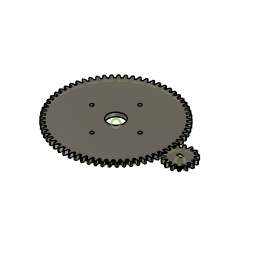
Gears v6 (Autodesk Fusion 360 design; units mm, degrees)
description: Spur Gear; Module: 2.0; Num Teeth: 15; Pressure Angle: 20.0; Backlash: 0.15 mm
description: Spur Gear; Module: 2.0; Num Teeth: 65; Pressure Angle: 20.0; Backlash: 0.15 mm
Autodesk Fusion 360 part; units mm, degrees
(part 1 of 8)
sketch "Sketch1" plane through (0, 0, 0) normal (0, 0, 1) x (1, 0, 0) in component "Spur Gear (15 teeth)"
  circle A0 centre (0, 0) radius 12.5492
extrude "Extrude1" add sketch "Sketch1" along normal blind 5 makes body 1 in component "Spur Gear (15 teeth)"
sketch "Sketch2" plane through (0, 0, 0) normal (0, 0, 1) x (1, 0, 0) in component "Spur Gear (15 teeth)"
  spline S0 degree 5 poles (13.9988, -1.6471) (14.0073, -1.6481) (14.0244, -1.6499) (14.05, -1.6517) (14.0843, -1.6528) (14.1272, -1.6522) (14.1702, -1.6502) (14.2133, -1.6473) (14.2564, -1.644) (14.2995, -1.6403) (14.3427, -1.6363) (14.3859, -1.6318) (14.4291, -1.6268) (14.4723, -1.621) (14.5156, -1.6146) (14.5589, -1.6075) (14.6022, -1.5999) (14.6454, -1.5918) (14.6887, -1.5833) (14.732, -1.5744) (14.7753, -1.5652) (14.8186, -1.5555) (14.8619, -1.5454) (14.9052, -1.5349) (14.9484, -1.524) (14.9917, -1.5126) (15.0349, -1.5009) (15.0782, -1.4887) (15.1214, -1.4762) (15.1646, -1.4634) (15.2077, -1.4502) (15.2509, -1.4366) (15.294, -1.4227) (15.3372, -1.4084) (15.3803, -1.3938) (15.4233, -1.3789) (15.4664, -1.3636) (15.5094, -1.348) (15.5524, -1.332) (15.5953, -1.3157) (15.6383, -1.2991) (15.6811, -1.2822) (15.724, -1.265) (15.7668, -1.2475) (15.8096, -1.2296) (15.8524, -1.2115) (15.8951, -1.193) (15.9378, -1.1743) (15.9804, -1.1552) (16.023, -1.1359) (16.0655, -1.1162) (16.108, -1.0963) (16.1505, -1.0761) (16.1929, -1.0556) (16.2353, -1.0348) (16.2776, -1.0137) (16.3199, -0.9924) (16.3621, -0.9707) (16.4043, -0.9488) (16.4464, -0.9266) (16.4885, -0.9042) (16.5305, -0.8814) (16.5725, -0.8584) (16.6144, -0.8351) (16.6562, -0.8116) (16.698, -0.7878) (16.7398, -0.7637) (16.7814, -0.7394) (16.8231, -0.7148) (16.8646, -0.6899) (16.9061, -0.6648) (16.9393, -0.6445) (16.9641, -0.6292) (16.9806, -0.6189) (16.9889, -0.6138) knots 0 0 0 0 0 0 0.01428571 0.02857143 0.04285714 0.05714286 0.07142857 0.08571429 0.1 0.11428571 0.12857143 0.14285714 0.15714286 0.17142857 0.18571429 0.2 0.21428571 0.22857143 0.24285714 0.25714286 0.27142857 0.28571429 0.3 0.31428571 0.32857143 0.34285714 0.35714286 0.37142857 0.38571429 0.4 0.41428571 0.42857143 0.44285714 0.45714286 0.47142857 0.48571429 0.5 0.51428571 0.52857143 0.54285714 0.55714286 0.57142857 0.58571429 0.6 0.61428571 0.62857143 0.64285714 0.65714286 0.67142857 0.68571429 0.7 0.71428571 0.72857143 0.74285714 0.75714286 0.77142857 0.78571429 0.8 0.81428571 0.82857143 0.84285714 0.85714286 0.87142857 0.88571429 0.9 0.91428571 0.92857143 0.94285714 0.95714286 0.97142857 0.98571429 1 1 1 1 1 1
  spline S1 degree 5 poles (13.9988, 1.6471) (14.0073, 1.6481) (14.0244, 1.6499) (14.05, 1.6517) (14.0843, 1.6528) (14.1272, 1.6522) (14.1702, 1.6502) (14.2133, 1.6473) (14.2564, 1.644) (14.2995, 1.6403) (14.3427, 1.6363) (14.3859, 1.6318) (14.4291, 1.6268) (14.4723, 1.621) (14.5156, 1.6146) (14.5589, 1.6075) (14.6022, 1.5999) (14.6454, 1.5918) (14.6887, 1.5833) (14.732, 1.5744) (14.7753, 1.5652) (14.8186, 1.5555) (14.8619, 1.5454) (14.9052, 1.5349) (14.9484, 1.524) (14.9917, 1.5126) (15.0349, 1.5009) (15.0782, 1.4887) (15.1214, 1.4762) (15.1646, 1.4634) (15.2077, 1.4502) (15.2509, 1.4366) (15.294, 1.4227) (15.3372, 1.4084) (15.3803, 1.3938) (15.4233, 1.3789) (15.4664, 1.3636) (15.5094, 1.348) (15.5524, 1.332) (15.5953, 1.3157) (15.6383, 1.2991) (15.6811, 1.2822) (15.724, 1.265) (15.7668, 1.2475) (15.8096, 1.2296) (15.8524, 1.2115) (15.8951, 1.193) (15.9378, 1.1743) (15.9804, 1.1552) (16.023, 1.1359) (16.0655, 1.1162) (16.108, 1.0963) (16.1505, 1.0761) (16.1929, 1.0556) (16.2353, 1.0348) (16.2776, 1.0137) (16.3199, 0.9924) (16.3621, 0.9707) (16.4043, 0.9488) (16.4464, 0.9266) (16.4885, 0.9042) (16.5305, 0.8814) (16.5725, 0.8584) (16.6144, 0.8351) (16.6562, 0.8116) (16.698, 0.7878) (16.7398, 0.7637) (16.7814, 0.7394) (16.8231, 0.7148) (16.8646, 0.6899) (16.9061, 0.6648) (16.9393, 0.6445) (16.9641, 0.6292) (16.9806, 0.6189) (16.9889, 0.6138) knots 0 0 0 0 0 0 0.01428571 0.02857143 0.04285714 0.05714286 0.07142857 0.08571429 0.1 0.11428571 0.12857143 0.14285714 0.15714286 0.17142857 0.18571429 0.2 0.21428571 0.22857143 0.24285714 0.25714286 0.27142857 0.28571429 0.3 0.31428571 0.32857143 0.34285714 0.35714286 0.37142857 0.38571429 0.4 0.41428571 0.42857143 0.44285714 0.45714286 0.47142857 0.48571429 0.5 0.51428571 0.52857143 0.54285714 0.55714286 0.57142857 0.58571429 0.6 0.61428571 0.62857143 0.64285714 0.65714286 0.67142857 0.68571429 0.7 0.71428571 0.72857143 0.74285714 0.75714286 0.77142857 0.78571429 0.8 0.81428571 0.82857143 0.84285714 0.85714286 0.87142857 0.88571429 0.9 0.91428571 0.92857143 0.94285714 0.95714286 0.97142857 0.98571429 1 1 1 1 1 1
  arc A0 (16.9889, -0.6138) -> (16.9889, 0.6138) centre (0, 0) ccw
  line L0 (12.4533, -1.4665) -> (13.9988, -1.6471)
  line L1 (12.4533, 1.4665) -> (13.9988, 1.6471)
  line L2 (12.4533, -1.4665) -> (12.4533, 1.4665)
  point P0 (14.2076, -1.6476)
  point P1 (14.4187, -1.6279)
  point P2 (14.6312, -1.5944)
  point P3 (14.8446, -1.5494)
  point P4 (15.0588, -1.4941)
  point P5 (15.2735, -1.4293)
  point P6 (15.4885, -1.3555)
  point P7 (15.7036, -1.2732)
  point P8 (15.9188, -1.1826)
  point P9 (16.1337, -1.084)
  point P10 (16.3484, -0.9777)
  point P11 (16.5625, -0.8638)
  point P12 (16.7761, -0.7424)
  point P13 (14.2076, 1.6476)
  point P14 (14.4187, 1.6279)
  point P15 (14.6312, 1.5944)
  point P16 (14.8446, 1.5494)
  point P17 (15.0588, 1.4941)
  point P18 (15.2735, 1.4293)
  point P19 (15.4885, 1.3555)
  point P20 (15.7036, 1.2732)
  point P21 (15.9188, 1.1826)
  point P22 (16.1337, 1.084)
  point P23 (16.3484, 0.9777)
  point P24 (16.5625, 0.8638)
  point P25 (16.7761, 0.7424)
extrude "Extrude2" add sketch "Sketch2" along normal blind 5 bodies 1 in component "Spur Gear (15 teeth)"
fillet "Fillet1" radius 1 2 edges at (12.4631, -1.4676, 2.5) (12.4631, 1.4676, 2.5) on bodies 1 in component "Spur Gear (15 teeth)"
pattern_circular "C-Pattern1" count 15 over 360 about axis through (0, 0, 0) along (0, 0, 1) of "Extrude2", "Fillet1" in component "Spur Gear (15 teeth)"
sketch "Sketch3" plane through (0, 0, 0) normal (0, 0, 1) x (1, 0, 0) in component "Spur Gear (15 teeth)"
  circle A0 centre (0, 0) radius 15 construction
sketch "Sketch1 (2)" plane through (0, 0, 0) normal (0, 0, 1) x (1, 0, 0) in component "Spur Gear (65 teeth)"
  circle A0 centre (0, 0) radius 62.5492
extrude "Extrude1'" add sketch "Sketch1 (2)" along normal blind 5 separate body makes body 2 in component "Spur Gear (65 teeth)"
sketch "Sketch2 (2)" plane through (0, 0, 0) normal (0, 0, 1) x (1, 0, 0) in component "Spur Gear (65 teeth)"
  spline S0 degree 5 poles (61.0348, -2.3506) (61.052, -2.3506) (61.0865, -2.3503) (61.1381, -2.3496) (61.2071, -2.3478) (61.2932, -2.3443) (61.3794, -2.3394) (61.4655, -2.3334) (61.5516, -2.3261) (61.6378, -2.3177) (61.7239, -2.3084) (61.81, -2.2982) (61.8961, -2.2872) (61.9822, -2.2755) (62.0683, -2.2632) (62.1543, -2.2502) (62.2403, -2.2367) (62.3263, -2.2225) (62.4122, -2.2076) (62.4982, -2.1922) (62.5841, -2.1761) (62.6699, -2.1595) (62.7558, -2.1424) (62.8416, -2.1247) (62.9274, -2.1065) (63.0131, -2.0878) (63.0988, -2.0687) (63.1845, -2.049) (63.2701, -2.0289) (63.3557, -2.0082) (63.4413, -1.9872) (63.5268, -1.9656) (63.6123, -1.9436) (63.6978, -1.9212) (63.7832, -1.8983) (63.8686, -1.875) (63.954, -1.8513) (64.0393, -1.8272) (64.1245, -1.8027) (64.2097, -1.7777) (64.2949, -1.7524) (64.3801, -1.7266) (64.4651, -1.7005) (64.5502, -1.674) (64.6352, -1.647) (64.7202, -1.6198) (64.8051, -1.5921) (64.89, -1.5641) (64.9748, -1.5357) (65.0596, -1.5069) (65.1443, -1.4778) (65.229, -1.4483) (65.3136, -1.4184) (65.3982, -1.3882) (65.4828, -1.3577) (65.5673, -1.3268) (65.6517, -1.2955) (65.7361, -1.264) (65.8205, -1.2321) (65.9047, -1.1998) (65.989, -1.1672) (66.0732, -1.1343) (66.1573, -1.1011) (66.2414, -1.0675) (66.3255, -1.0336) (66.4094, -0.9994) (66.4934, -0.9649) (66.5772, -0.93) (66.6611, -0.8949) (66.7448, -0.8594) (66.8285, -0.8236) (66.8955, -0.7947) (66.9456, -0.7729) (66.9791, -0.7583) (66.9958, -0.751) knots 0 0 0 0 0 0 0.01428571 0.02857143 0.04285714 0.05714286 0.07142857 0.08571429 0.1 0.11428571 0.12857143 0.14285714 0.15714286 0.17142857 0.18571429 0.2 0.21428571 0.22857143 0.24285714 0.25714286 0.27142857 0.28571429 0.3 0.31428571 0.32857143 0.34285714 0.35714286 0.37142857 0.38571429 0.4 0.41428571 0.42857143 0.44285714 0.45714286 0.47142857 0.48571429 0.5 0.51428571 0.52857143 0.54285714 0.55714286 0.57142857 0.58571429 0.6 0.61428571 0.62857143 0.64285714 0.65714286 0.67142857 0.68571429 0.7 0.71428571 0.72857143 0.74285714 0.75714286 0.77142857 0.78571429 0.8 0.81428571 0.82857143 0.84285714 0.85714286 0.87142857 0.88571429 0.9 0.91428571 0.92857143 0.94285714 0.95714286 0.97142857 0.98571429 1 1 1 1 1 1
  spline S1 degree 5 poles (61.0348, 2.3506) (61.052, 2.3506) (61.0865, 2.3503) (61.1381, 2.3496) (61.2071, 2.3478) (61.2932, 2.3443) (61.3794, 2.3394) (61.4655, 2.3334) (61.5516, 2.3261) (61.6378, 2.3177) (61.7239, 2.3084) (61.81, 2.2982) (61.8961, 2.2872) (61.9822, 2.2755) (62.0683, 2.2632) (62.1543, 2.2502) (62.2403, 2.2367) (62.3263, 2.2225) (62.4122, 2.2076) (62.4982, 2.1922) (62.5841, 2.1761) (62.6699, 2.1595) (62.7558, 2.1424) (62.8416, 2.1247) (62.9274, 2.1065) (63.0131, 2.0878) (63.0988, 2.0687) (63.1845, 2.049) (63.2701, 2.0289) (63.3557, 2.0082) (63.4413, 1.9872) (63.5268, 1.9656) (63.6123, 1.9436) (63.6978, 1.9212) (63.7832, 1.8983) (63.8686, 1.875) (63.954, 1.8513) (64.0393, 1.8272) (64.1245, 1.8027) (64.2097, 1.7777) (64.2949, 1.7524) (64.3801, 1.7266) (64.4651, 1.7005) (64.5502, 1.674) (64.6352, 1.647) (64.7202, 1.6198) (64.8051, 1.5921) (64.89, 1.5641) (64.9748, 1.5357) (65.0596, 1.5069) (65.1443, 1.4778) (65.229, 1.4483) (65.3136, 1.4184) (65.3982, 1.3882) (65.4828, 1.3577) (65.5673, 1.3268) (65.6517, 1.2955) (65.7361, 1.264) (65.8205, 1.2321) (65.9047, 1.1998) (65.989, 1.1672) (66.0732, 1.1343) (66.1573, 1.1011) (66.2414, 1.0675) (66.3255, 1.0336) (66.4094, 0.9994) (66.4934, 0.9649) (66.5772, 0.93) (66.6611, 0.8949) (66.7448, 0.8594) (66.8285, 0.8236) (66.8955, 0.7947) (66.9456, 0.7729) (66.9791, 0.7583) (66.9958, 0.751) knots 0 0 0 0 0 0 0.01428571 0.02857143 0.04285714 0.05714286 0.07142857 0.08571429 0.1 0.11428571 0.12857143 0.14285714 0.15714286 0.17142857 0.18571429 0.2 0.21428571 0.22857143 0.24285714 0.25714286 0.27142857 0.28571429 0.3 0.31428571 0.32857143 0.34285714 0.35714286 0.37142857 0.38571429 0.4 0.41428571 0.42857143 0.44285714 0.45714286 0.47142857 0.48571429 0.5 0.51428571 0.52857143 0.54285714 0.55714286 0.57142857 0.58571429 0.6 0.61428571 0.62857143 0.64285714 0.65714286 0.67142857 0.68571429 0.7 0.71428571 0.72857143 0.74285714 0.75714286 0.77142857 0.78571429 0.8 0.81428571 0.82857143 0.84285714 0.85714286 0.87142857 0.88571429 0.9 0.91428571 0.92857143 0.94285714 0.95714286 0.97142857 0.98571429 1 1 1 1 1 1
  arc A0 (66.9958, -0.751) -> (66.9958, 0.751) centre (0, 0) ccw
  line L0 (61.0348, 2.3506) -> (61.0348, -2.3506)
  point P0 (61.4586, -2.3336)
  point P1 (61.8834, -2.2887)
  point P2 (62.3089, -2.2252)
  point P3 (62.7347, -2.1465)
  point P4 (63.1609, -2.0543)
  point P5 (63.5873, -1.95)
  point P6 (64.0137, -1.8344)
  point P7 (64.4402, -1.7081)
  point P8 (64.8667, -1.5717)
  point P9 (65.293, -1.4256)
  point P10 (65.7192, -1.2702)
  point P11 (66.145, -1.1059)
  point P12 (66.5706, -0.9327)
  point P13 (61.4586, 2.3336)
  point P14 (61.8834, 2.2887)
  point P15 (62.3089, 2.2252)
  point P16 (62.7347, 2.1465)
  point P17 (63.1609, 2.0543)
  point P18 (63.5873, 1.95)
  point P19 (64.0137, 1.8344)
  point P20 (64.4402, 1.7081)
  point P21 (64.8667, 1.5717)
  point P22 (65.293, 1.4256)
  point P23 (65.7192, 1.2702)
  point P24 (66.145, 1.1059)
  point P25 (66.5706, 0.9327)
extrude "Extrude2'" add sketch "Sketch2 (2)" along normal blind 5 bodies 2 in component "Spur Gear (65 teeth)"
fillet "Fillet1'" radius 0.2 2 edges at (62.5109, 2.1897, 2.5) (62.5109, -2.1897, 2.5) on bodies 2 in component "Spur Gear (65 teeth)"
pattern_circular "C-Pattern1'" count 65 over 360 about axis through (0, 0, 0) along (0, 0, 1) of "Extrude2'", "Fillet1'" in component "Spur Gear (65 teeth)"
sketch "Sketch3 (2)" plane through (0, 0, 0) normal (0, 0, 1) x (1, 0, 0) in component "Spur Gear (65 teeth)"
  circle A0 centre (0, 0) radius 65 construction
sketch "Sketch1 (3)" plane through (0, 0, 5) normal (0, 0, 1) x (-1, 0, 0)
  arc A0 (-92.2249, 2.8347) -> (-92.3209, 2.3827) centre (-80, 0) ccw
  arc A1 (-93.4188, 1.5793) -> (-92.3209, 2.3827) centre (-93.3027, 2.5726) ccw
  line L0 (-93.4188, 1.5793) -> (-93.9988, 1.6471)
  line L1 (-93.9988, -1.6471) -> (-93.4188, -1.5793)
  arc A2 (-92.3209, -2.3827) -> (-93.4188, -1.5793) centre (-93.3027, -2.5726) ccw
  arc A3 (-92.9011, -4.0151) -> (-92.2249, -2.8347) centre (-93.199, -3.0605) ccw
  line L2 (-92.9011, -4.0151) -> (-93.4585, -4.1891)
  line L3 (-92.1186, -7.1986) -> (-91.6164, -6.9007)
  arc A4 (-90.2866, -7.1881) -> (-91.6164, -6.9007) centre (-91.1063, -7.7609) ccw
  arc A5 (-90.1526, -8.9154) -> (-90.015, -7.5619) centre (-90.8131, -8.1645) ccw
  line L4 (-90.1526, -8.9154) -> (-90.5911, -9.301)
  line L5 (-88.143, -11.5053) -> (-87.8053, -11.0289)
  arc A6 (-86.4736, -10.7506) -> (-87.8053, -11.0289) centre (-86.9895, -11.6072) ccw
  arc A7 (-85.6487, -12.274) -> (-86.0735, -10.9816) centre (-86.5574, -11.8567) ccw
  line L6 (-85.6487, -12.274) -> (-85.8924, -12.8047)
  line L7 (-82.7594, -13.8227) -> (-82.6446, -13.2501)
  arc A8 (-81.5413, -12.4542) -> (-82.6446, -13.2501) centre (-81.6641, -13.4466) ccw
  arc A9 (-80.168, -13.5104) -> (-81.0818, -12.5025) centre (-81.168, -13.4988) ccw
  line L8 (-80.168, -13.5104) -> (-80.1748, -14.0943)
  line L9 (-76.8986, -13.75) -> (-77.0267, -13.1803)
  arc A10 (-76.3425, -12.0044) -> (-77.0267, -13.1803) centre (-76.051, -12.961) ccw
  arc A11 (-74.6583, -12.4107) -> (-75.903, -11.8616) centre (-75.5765, -12.8068) ccw
  line L10 (-74.6583, -12.4107) -> (-74.4271, -12.9469)
  line L11 (-71.5741, -11.2998) -> (-71.9228, -10.8314)
  arc A12 (-71.7761, -9.4789) -> (-71.9228, -10.8314) centre (-71.1207, -10.2342) ccw
  arc A13 (-70.0722, -9.1651) -> (-71.4327, -9.1697) centre (-70.75, -9.9004) ccw
  line L12 (-70.0722, -9.1651) -> (-69.6429, -9.5609)
  line L13 (-67.7066, -6.8957) -> (-68.2156, -6.6097)
  arc A14 (-68.6316, -5.3144) -> (-68.2156, -6.6097) centre (-67.7257, -5.7379) ccw
  arc A15 (-67.2027, -4.3348) -> (-68.4437, -4.8923) centre (-67.5228, -5.2821) ccw
  line L14 (-67.2027, -4.3348) -> (-66.6495, -4.5217)
  line L15 (-65.9646, -1.2994) -> (-66.546, -1.2451)
  arc A16 (-67.4529, -0.231) -> (-66.546, -1.2451) centre (-66.4531, -0.2494) ccw
  arc A17 (-66.546, 1.2451) -> (-67.4529, 0.231) centre (-66.4531, 0.2494) ccw
  line L16 (-66.546, 1.2451) -> (-65.9646, 1.2994)
  line L17 (-66.6495, 4.5217) -> (-67.2027, 4.3348)
  arc A18 (-68.4437, 4.8923) -> (-67.2027, 4.3348) centre (-67.5228, 5.2821) ccw
  arc A19 (-68.2156, 6.6097) -> (-68.6316, 5.3144) centre (-67.7257, 5.7379) ccw
  line L18 (-68.2156, 6.6097) -> (-67.7066, 6.8957)
  line L19 (-69.6429, 9.5609) -> (-70.0722, 9.1651)
  arc A20 (-71.4327, 9.1697) -> (-70.0722, 9.1651) centre (-70.75, 9.9004) ccw
  arc A21 (-71.9228, 10.8314) -> (-71.7761, 9.4789) centre (-71.1207, 10.2342) ccw
  line L20 (-71.9228, 10.8314) -> (-71.5741, 11.2998)
  line L21 (-74.4271, 12.9469) -> (-74.6583, 12.4107)
  arc A22 (-75.903, 11.8616) -> (-74.6583, 12.4107) centre (-75.5765, 12.8068) ccw
  arc A23 (-77.0267, 13.1803) -> (-76.3425, 12.0044) centre (-76.051, 12.961) ccw
  line L22 (-77.0267, 13.1803) -> (-76.8986, 13.75)
  line L23 (-80.1748, 14.0943) -> (-80.168, 13.5104)
  arc A24 (-81.0818, 12.5025) -> (-80.168, 13.5104) centre (-81.168, 13.4988) ccw
  arc A25 (-82.6446, 13.2501) -> (-81.5413, 12.4542) centre (-81.6641, 13.4466) ccw
  line L24 (-82.6446, 13.2501) -> (-82.7594, 13.8227)
  line L25 (-85.8924, 12.8047) -> (-85.6487, 12.274)
  arc A26 (-86.0735, 10.9816) -> (-85.6487, 12.274) centre (-86.5574, 11.8567) ccw
  arc A27 (-87.8053, 11.0289) -> (-86.4736, 10.7506) centre (-86.9895, 11.6072) ccw
  line L26 (-87.8053, 11.0289) -> (-88.143, 11.5053)
  line L27 (-90.5911, 9.301) -> (-90.1526, 8.9154)
  arc A28 (-90.015, 7.5619) -> (-90.1526, 8.9154) centre (-90.8131, 8.1645) ccw
  arc A29 (-91.6164, 6.9007) -> (-90.2866, 7.1881) centre (-91.1063, 7.7609) ccw
  line L28 (-91.6164, 6.9007) -> (-92.1186, 7.1986)
  line L29 (-93.4585, 4.1891) -> (-92.9011, 4.0151)
  arc A30 (-92.2249, 2.8347) -> (-92.9011, 4.0151) centre (-93.199, 3.0605) ccw
  line L30 (-77.35, -1.65) -> (-82.65, -1.65)
  line L31 (-82.65, -1.65) -> (-82.65, 1.65)
  line L32 (-82.65, 1.65) -> (-77.35, 1.65)
  line L33 (-77.35, 1.65) -> (-77.35, -1.65)
  line L34 (-77.35, -1.65) -> (-82.65, 1.65) construction
  line L35 (-82.65, -1.65) -> (-77.35, 1.65) construction
  spline S0 degree 5 poles (-93.9988, 1.6471) (-94.0073, 1.6481) (-94.0244, 1.6499) (-94.05, 1.6517) (-94.0843, 1.6528) (-94.1272, 1.6522) (-94.1702, 1.6502) (-94.2133, 1.6473) (-94.2564, 1.644) (-94.2995, 1.6403) (-94.3427, 1.6363) (-94.3859, 1.6318) (-94.4291, 1.6268) (-94.4723, 1.621) (-94.5156, 1.6146) (-94.5589, 1.6075) (-94.6022, 1.5999) (-94.6454, 1.5918) (-94.6887, 1.5833) (-94.732, 1.5744) (-94.7753, 1.5652) (-94.8186, 1.5555) (-94.8619, 1.5454) (-94.9052, 1.5349) (-94.9484, 1.524) (-94.9917, 1.5126) (-95.0349, 1.5009) (-95.0782, 1.4887) (-95.1214, 1.4762) (-95.1646, 1.4634) (-95.2077, 1.4502) (-95.2509, 1.4366) (-95.294, 1.4227) (-95.3372, 1.4084) (-95.3803, 1.3938) (-95.4233, 1.3789) (-95.4664, 1.3636) (-95.5094, 1.348) (-95.5524, 1.332) (-95.5953, 1.3157) (-95.6383, 1.2991) (-95.6811, 1.2822) (-95.724, 1.265) (-95.7668, 1.2475) (-95.8096, 1.2296) (-95.8524, 1.2115) (-95.8951, 1.193) (-95.9378, 1.1743) (-95.9804, 1.1552) (-96.023, 1.1359) (-96.0655, 1.1162) (-96.108, 1.0963) (-96.1505, 1.0761) (-96.1929, 1.0556) (-96.2353, 1.0348) (-96.2776, 1.0137) (-96.3199, 0.9924) (-96.3621, 0.9707) (-96.4043, 0.9488) (-96.4464, 0.9266) (-96.4885, 0.9042) (-96.5305, 0.8814) (-96.5725, 0.8584) (-96.6144, 0.8351) (-96.6562, 0.8116) (-96.698, 0.7878) (-96.7398, 0.7637) (-96.7814, 0.7394) (-96.8231, 0.7148) (-96.8646, 0.6899) (-96.9061, 0.6648) (-96.9393, 0.6445) (-96.9641, 0.6292) (-96.9806, 0.6189) (-96.9889, 0.6138) knots 0 0 0 0 0 0 0.01428571 0.02857143 0.04285714 0.05714286 0.07142857 0.08571429 0.1 0.11428571 0.12857143 0.14285714 0.15714286 0.17142857 0.18571429 0.2 0.21428571 0.22857143 0.24285714 0.25714286 0.27142857 0.28571429 0.3 0.31428571 0.32857143 0.34285714 0.35714286 0.37142857 0.38571429 0.4 0.41428571 0.42857143 0.44285714 0.45714286 0.47142857 0.48571429 0.5 0.51428571 0.52857143 0.54285714 0.55714286 0.57142857 0.58571429 0.6 0.61428571 0.62857143 0.64285714 0.65714286 0.67142857 0.68571429 0.7 0.71428571 0.72857143 0.74285714 0.75714286 0.77142857 0.78571429 0.8 0.81428571 0.82857143 0.84285714 0.85714286 0.87142857 0.88571429 0.9 0.91428571 0.92857143 0.94285714 0.95714286 0.97142857 0.98571429 1 1 1 1 1 1
  arc A31 (-96.9889, 0.6138) -> (-96.9889, -0.6138) centre (-80, 0) ccw
  spline S1 degree 5 poles (-96.9889, -0.6138) (-96.9806, -0.6189) (-96.9641, -0.6292) (-96.9393, -0.6445) (-96.9061, -0.6648) (-96.8646, -0.6899) (-96.8231, -0.7148) (-96.7814, -0.7394) (-96.7398, -0.7637) (-96.698, -0.7878) (-96.6562, -0.8116) (-96.6144, -0.8351) (-96.5725, -0.8584) (-96.5305, -0.8814) (-96.4885, -0.9042) (-96.4464, -0.9266) (-96.4043, -0.9488) (-96.3621, -0.9707) (-96.3199, -0.9924) (-96.2776, -1.0137) (-96.2353, -1.0348) (-96.1929, -1.0556) (-96.1505, -1.0761) (-96.108, -1.0963) (-96.0655, -1.1162) (-96.023, -1.1359) (-95.9804, -1.1552) (-95.9378, -1.1743) (-95.8951, -1.193) (-95.8524, -1.2115) (-95.8096, -1.2296) (-95.7668, -1.2475) (-95.724, -1.265) (-95.6811, -1.2822) (-95.6383, -1.2991) (-95.5953, -1.3157) (-95.5524, -1.332) (-95.5094, -1.348) (-95.4664, -1.3636) (-95.4233, -1.3789) (-95.3803, -1.3938) (-95.3372, -1.4084) (-95.294, -1.4227) (-95.2509, -1.4366) (-95.2077, -1.4502) (-95.1646, -1.4634) (-95.1214, -1.4762) (-95.0782, -1.4887) (-95.0349, -1.5009) (-94.9917, -1.5126) (-94.9484, -1.524) (-94.9052, -1.5349) (-94.8619, -1.5454) (-94.8186, -1.5555) (-94.7753, -1.5652) (-94.732, -1.5744) (-94.6887, -1.5833) (-94.6454, -1.5918) (-94.6022, -1.5999) (-94.5589, -1.6075) (-94.5156, -1.6146) (-94.4723, -1.621) (-94.4291, -1.6268) (-94.3859, -1.6318) (-94.3427, -1.6363) (-94.2995, -1.6403) (-94.2564, -1.644) (-94.2133, -1.6473) (-94.1702, -1.6502) (-94.1272, -1.6522) (-94.0843, -1.6528) (-94.05, -1.6517) (-94.0244, -1.6499) (-94.0073, -1.6481) (-93.9988, -1.6471) knots -1 -1 -1 -1 -1 -1 -0.98571429 -0.97142857 -0.95714286 -0.94285714 -0.92857143 -0.91428571 -0.9 -0.88571429 -0.87142857 -0.85714286 -0.84285714 -0.82857143 -0.81428571 -0.8 -0.78571429 -0.77142857 -0.75714286 -0.74285714 -0.72857143 -0.71428571 -0.7 -0.68571429 -0.67142857 -0.65714286 -0.64285714 -0.62857143 -0.61428571 -0.6 -0.58571429 -0.57142857 -0.55714286 -0.54285714 -0.52857143 -0.51428571 -0.5 -0.48571429 -0.47142857 -0.45714286 -0.44285714 -0.42857143 -0.41428571 -0.4 -0.38571429 -0.37142857 -0.35714286 -0.34285714 -0.32857143 -0.31428571 -0.3 -0.28571429 -0.27142857 -0.25714286 -0.24285714 -0.22857143 -0.21428571 -0.2 -0.18571429 -0.17142857 -0.15714286 -0.14285714 -0.12857143 -0.11428571 -0.1 -0.08571429 -0.07142857 -0.05714286 -0.04285714 -0.02857143 -0.01428571 0 0 0 0 0 0
  arc A32 (-92.3209, -2.3827) -> (-92.2249, -2.8347) centre (-80, 0) ccw
  spline S2 degree 5 poles (-93.4585, -4.1891) (-93.4667, -4.1917) (-93.483, -4.197) (-93.5072, -4.2057) (-93.5389, -4.2187) (-93.5778, -4.2367) (-93.6163, -4.256) (-93.6545, -4.2761) (-93.6925, -4.2967) (-93.7304, -4.3176) (-93.7682, -4.3389) (-93.8059, -4.3605) (-93.8433, -4.3827) (-93.8805, -4.4056) (-93.9174, -4.429) (-93.954, -4.4531) (-93.9905, -4.4777) (-94.0267, -4.5027) (-94.0628, -4.528) (-94.0988, -4.5537) (-94.1345, -4.5798) (-94.1702, -4.6062) (-94.2056, -4.633) (-94.2408, -4.6602) (-94.2759, -4.6878) (-94.3108, -4.7158) (-94.3455, -4.7442) (-94.3801, -4.7728) (-94.4145, -4.8018) (-94.4487, -4.8311) (-94.4828, -4.8608) (-94.5167, -4.8907) (-94.5505, -4.9209) (-94.5841, -4.9515) (-94.6175, -4.9824) (-94.6507, -5.0136) (-94.6838, -5.0451) (-94.7168, -5.0768) (-94.7496, -5.1089) (-94.7822, -5.1412) (-94.8147, -5.1738) (-94.847, -5.2067) (-94.8791, -5.2399) (-94.9111, -5.2733) (-94.9429, -5.307) (-94.9746, -5.341) (-95.0061, -5.3752) (-95.0375, -5.4097) (-95.0687, -5.4444) (-95.0997, -5.4794) (-95.1306, -5.5147) (-95.1613, -5.5502) (-95.1919, -5.5859) (-95.2223, -5.6219) (-95.2526, -5.6582) (-95.2827, -5.6946) (-95.3126, -5.7313) (-95.3424, -5.7683) (-95.372, -5.8054) (-95.4014, -5.8428) (-95.4307, -5.8805) (-95.4599, -5.9183) (-95.4888, -5.9564) (-95.5177, -5.9947) (-95.5463, -6.0333) (-95.5748, -6.072) (-95.6032, -6.111) (-95.6313, -6.1502) (-95.6594, -6.1896) (-95.6872, -6.2292) (-95.7149, -6.269) (-95.7369, -6.301) (-95.7534, -6.3251) (-95.7643, -6.3412) (-95.7698, -6.3493) knots 0 0 0 0 0 0 0.01428571 0.02857143 0.04285714 0.05714286 0.07142857 0.08571429 0.1 0.11428571 0.12857143 0.14285714 0.15714286 0.17142857 0.18571429 0.2 0.21428571 0.22857143 0.24285714 0.25714286 0.27142857 0.28571429 0.3 0.31428571 0.32857143 0.34285714 0.35714286 0.37142857 0.38571429 0.4 0.41428571 0.42857143 0.44285714 0.45714286 0.47142857 0.48571429 0.5 0.51428571 0.52857143 0.54285714 0.55714286 0.57142857 0.58571429 0.6 0.61428571 0.62857143 0.64285714 0.65714286 0.67142857 0.68571429 0.7 0.71428571 0.72857143 0.74285714 0.75714286 0.77142857 0.78571429 0.8 0.81428571 0.82857143 0.84285714 0.85714286 0.87142857 0.88571429 0.9 0.91428571 0.92857143 0.94285714 0.95714286 0.97142857 0.98571429 1 1 1 1 1 1
  arc A33 (-95.7698, -6.3493) -> (-95.2705, -7.4707) centre (-80, 0) ccw
  spline S3 degree 5 poles (-95.2705, -7.4707) (-95.2609, -7.4721) (-95.2416, -7.4747) (-95.2126, -7.4786) (-95.1741, -7.4837) (-95.126, -7.4897) (-95.0779, -7.4955) (-95.0299, -7.5011) (-94.9819, -7.5064) (-94.934, -7.5114) (-94.8861, -7.5161) (-94.8383, -7.5206) (-94.7906, -7.5248) (-94.7429, -7.5288) (-94.6952, -7.5325) (-94.6477, -7.5359) (-94.6001, -7.539) (-94.5527, -7.5419) (-94.5053, -7.5445) (-94.458, -7.5468) (-94.4108, -7.5488) (-94.3636, -7.5506) (-94.3165, -7.5521) (-94.2695, -7.5533) (-94.2226, -7.5542) (-94.1757, -7.5548) (-94.1289, -7.5552) (-94.0822, -7.5552) (-94.0356, -7.555) (-93.9891, -7.5545) (-93.9427, -7.5537) (-93.8963, -7.5526) (-93.8501, -7.5512) (-93.8039, -7.5495) (-93.7578, -7.5475) (-93.7119, -7.5452) (-93.666, -7.5426) (-93.6203, -7.5397) (-93.5746, -7.5364) (-93.5291, -7.5329) (-93.4836, -7.529) (-93.4383, -7.5249) (-93.3931, -7.5204) (-93.3481, -7.5155) (-93.3031, -7.5103) (-93.2583, -7.5048) (-93.2136, -7.499) (-93.1691, -7.4929) (-93.1246, -7.4864) (-93.0803, -7.4795) (-93.0362, -7.4723) (-92.9922, -7.4647) (-92.9484, -7.4567) (-92.9048, -7.4483) (-92.8613, -7.4395) (-92.818, -7.4304) (-92.7748, -7.4209) (-92.7318, -7.411) (-92.689, -7.4008) (-92.6464, -7.3902) (-92.604, -7.379) (-92.5618, -7.3673) (-92.52, -7.355) (-92.4784, -7.342) (-92.4372, -7.3285) (-92.3961, -7.3146) (-92.3552, -7.3005) (-92.3144, -7.286) (-92.2739, -7.2711) (-92.2338, -7.2554) (-92.1943, -7.2385) (-92.1635, -7.2236) (-92.1409, -7.2115) (-92.126, -7.2029) (-92.1186, -7.1986) knots -1 -1 -1 -1 -1 -1 -0.98571429 -0.97142857 -0.95714286 -0.94285714 -0.92857143 -0.91428571 -0.9 -0.88571429 -0.87142857 -0.85714286 -0.84285714 -0.82857143 -0.81428571 -0.8 -0.78571429 -0.77142857 -0.75714286 -0.74285714 -0.72857143 -0.71428571 -0.7 -0.68571429 -0.67142857 -0.65714286 -0.64285714 -0.62857143 -0.61428571 -0.6 -0.58571429 -0.57142857 -0.55714286 -0.54285714 -0.52857143 -0.51428571 -0.5 -0.48571429 -0.47142857 -0.45714286 -0.44285714 -0.42857143 -0.41428571 -0.4 -0.38571429 -0.37142857 -0.35714286 -0.34285714 -0.32857143 -0.31428571 -0.3 -0.28571429 -0.27142857 -0.25714286 -0.24285714 -0.22857143 -0.21428571 -0.2 -0.18571429 -0.17142857 -0.15714286 -0.14285714 -0.12857143 -0.11428571 -0.1 -0.08571429 -0.07142857 -0.05714286 -0.04285714 -0.02857143 -0.01428571 0 0 0 0 0 0
  arc A34 (-90.2866, -7.1881) -> (-90.015, -7.5619) centre (-80, 0) ccw
  spline S4 degree 5 poles (-90.5911, -9.301) (-90.5975, -9.3067) (-90.6102, -9.3182) (-90.6288, -9.336) (-90.6525, -9.3607) (-90.6808, -9.393) (-90.7081, -9.4263) (-90.7347, -9.4602) (-90.7611, -9.4945) (-90.7872, -9.529) (-90.8131, -9.5638) (-90.8387, -9.5989) (-90.8639, -9.6344) (-90.8885, -9.6704) (-90.9127, -9.7068) (-90.9364, -9.7437) (-90.9597, -9.781) (-90.9827, -9.8186) (-91.0053, -9.8564) (-91.0277, -9.8945) (-91.0498, -9.9329) (-91.0716, -9.9715) (-91.093, -10.0104) (-91.1142, -10.0496) (-91.135, -10.0891) (-91.1555, -10.1289) (-91.1757, -10.1689) (-91.1956, -10.2091) (-91.2152, -10.2496) (-91.2346, -10.2903) (-91.2537, -10.3312) (-91.2725, -10.3724) (-91.291, -10.4137) (-91.3092, -10.4553) (-91.3272, -10.4971) (-91.3449, -10.5391) (-91.3624, -10.5813) (-91.3795, -10.6238) (-91.3964, -10.6664) (-91.4131, -10.7092) (-91.4295, -10.7522) (-91.4456, -10.7954) (-91.4615, -10.8387) (-91.4771, -10.8823) (-91.4925, -10.926) (-91.5076, -10.97) (-91.5225, -11.014) (-91.5371, -11.0583) (-91.5515, -11.1027) (-91.5656, -11.1473) (-91.5795, -11.1921) (-91.5931, -11.237) (-91.6065, -11.2821) (-91.6196, -11.3274) (-91.6325, -11.3728) (-91.6452, -11.4183) (-91.6576, -11.464) (-91.6698, -11.5099) (-91.6817, -11.5559) (-91.6934, -11.602) (-91.7049, -11.6483) (-91.7161, -11.6948) (-91.7271, -11.7413) (-91.7378, -11.7881) (-91.7483, -11.8349) (-91.7586, -11.8819) (-91.7686, -11.929) (-91.7784, -11.9763) (-91.788, -12.0237) (-91.7974, -12.0712) (-91.8065, -12.1188) (-91.8136, -12.1571) (-91.8188, -12.1858) (-91.8222, -12.2049) (-91.8239, -12.2145) knots 0 0 0 0 0 0 0.01428571 0.02857143 0.04285714 0.05714286 0.07142857 0.08571429 0.1 0.11428571 0.12857143 0.14285714 0.15714286 0.17142857 0.18571429 0.2 0.21428571 0.22857143 0.24285714 0.25714286 0.27142857 0.28571429 0.3 0.31428571 0.32857143 0.34285714 0.35714286 0.37142857 0.38571429 0.4 0.41428571 0.42857143 0.44285714 0.45714286 0.47142857 0.48571429 0.5 0.51428571 0.52857143 0.54285714 0.55714286 0.57142857 0.58571429 0.6 0.61428571 0.62857143 0.64285714 0.65714286 0.67142857 0.68571429 0.7 0.71428571 0.72857143 0.74285714 0.75714286 0.77142857 0.78571429 0.8 0.81428571 0.82857143 0.84285714 0.85714286 0.87142857 0.88571429 0.9 0.91428571 0.92857143 0.94285714 0.95714286 0.97142857 0.98571429 1 1 1 1 1 1
  arc A35 (-91.8239, -12.2145) -> (-90.9117, -13.0359) centre (-80, 0) ccw
  spline S5 degree 5 poles (-90.9117, -13.0359) (-90.9023, -13.0332) (-90.8836, -13.0278) (-90.8556, -13.0196) (-90.8183, -13.0085) (-90.7719, -12.9945) (-90.7256, -12.9803) (-90.6795, -12.9658) (-90.6335, -12.9511) (-90.5877, -12.9362) (-90.5421, -12.9211) (-90.4966, -12.9057) (-90.4512, -12.8901) (-90.406, -12.8743) (-90.361, -12.8583) (-90.3162, -12.8421) (-90.2715, -12.8256) (-90.227, -12.809) (-90.1827, -12.7921) (-90.1385, -12.7749) (-90.0945, -12.7576) (-90.0507, -12.74) (-90.0071, -12.7222) (-89.9637, -12.7042) (-89.9204, -12.6859) (-89.8773, -12.6675) (-89.8345, -12.6487) (-89.7918, -12.6298) (-89.7493, -12.6106) (-89.707, -12.5913) (-89.6649, -12.5716) (-89.623, -12.5518) (-89.5813, -12.5317) (-89.5398, -12.5113) (-89.4986, -12.4908) (-89.4575, -12.47) (-89.4167, -12.4489) (-89.3761, -12.4277) (-89.3357, -12.4062) (-89.2955, -12.3844) (-89.2556, -12.3624) (-89.2159, -12.3402) (-89.1764, -12.3177) (-89.1372, -12.2949) (-89.0983, -12.2719) (-89.0596, -12.2487) (-89.0211, -12.2252) (-88.9829, -12.2014) (-88.945, -12.1774) (-88.9073, -12.1531) (-88.8699, -12.1286) (-88.8328, -12.1038) (-88.796, -12.0786) (-88.7596, -12.0532) (-88.7235, -12.0275) (-88.6876, -12.0015) (-88.6521, -11.9753) (-88.6168, -11.9488) (-88.5818, -11.922) (-88.5472, -11.895) (-88.513, -11.8676) (-88.4792, -11.8397) (-88.446, -11.8114) (-88.4134, -11.7827) (-88.3811, -11.7536) (-88.3493, -11.7242) (-88.3177, -11.6946) (-88.2863, -11.6648) (-88.2554, -11.6347) (-88.2251, -11.6041) (-88.1959, -11.5726) (-88.1738, -11.5464) (-88.1581, -11.5261) (-88.1479, -11.5123) (-88.143, -11.5053) knots -1 -1 -1 -1 -1 -1 -0.98571429 -0.97142857 -0.95714286 -0.94285714 -0.92857143 -0.91428571 -0.9 -0.88571429 -0.87142857 -0.85714286 -0.84285714 -0.82857143 -0.81428571 -0.8 -0.78571429 -0.77142857 -0.75714286 -0.74285714 -0.72857143 -0.71428571 -0.7 -0.68571429 -0.67142857 -0.65714286 -0.64285714 -0.62857143 -0.61428571 -0.6 -0.58571429 -0.57142857 -0.55714286 -0.54285714 -0.52857143 -0.51428571 -0.5 -0.48571429 -0.47142857 -0.45714286 -0.44285714 -0.42857143 -0.41428571 -0.4 -0.38571429 -0.37142857 -0.35714286 -0.34285714 -0.32857143 -0.31428571 -0.3 -0.28571429 -0.27142857 -0.25714286 -0.24285714 -0.22857143 -0.21428571 -0.2 -0.18571429 -0.17142857 -0.15714286 -0.14285714 -0.12857143 -0.11428571 -0.1 -0.08571429 -0.07142857 -0.05714286 -0.04285714 -0.02857143 -0.01428571 0 0 0 0 0 0
  arc A36 (-86.4736, -10.7506) -> (-86.0735, -10.9816) centre (-80, 0) ccw
  spline S6 degree 5 poles (-85.8924, -12.8047) (-85.896, -12.8125) (-85.9029, -12.8282) (-85.9126, -12.8519) (-85.9242, -12.8842) (-85.9369, -12.9252) (-85.9483, -12.9667) (-85.9589, -13.0086) (-85.969, -13.0506) (-85.9788, -13.0928) (-85.9883, -13.1351) (-85.9974, -13.1775) (-86.006, -13.2202) (-86.0139, -13.2631) (-86.0211, -13.3062) (-86.0278, -13.3496) (-86.0339, -13.3931) (-86.0396, -13.4368) (-86.0449, -13.4805) (-86.0498, -13.5245) (-86.0544, -13.5685) (-86.0586, -13.6126) (-86.0624, -13.6569) (-86.0657, -13.7013) (-86.0687, -13.7459) (-86.0713, -13.7905) (-86.0734, -13.8353) (-86.0753, -13.8801) (-86.0767, -13.9251) (-86.0779, -13.9702) (-86.0786, -14.0153) (-86.0791, -14.0605) (-86.0792, -14.1059) (-86.0789, -14.1513) (-86.0784, -14.1968) (-86.0775, -14.2424) (-86.0762, -14.288) (-86.0746, -14.3338) (-86.0728, -14.3796) (-86.0706, -14.4255) (-86.068, -14.4714) (-86.0652, -14.5174) (-86.0621, -14.5635) (-86.0586, -14.6096) (-86.0549, -14.6559) (-86.0509, -14.7021) (-86.0465, -14.7484) (-86.0419, -14.7948) (-86.0369, -14.8413) (-86.0317, -14.8877) (-86.0261, -14.9343) (-86.0203, -14.9809) (-86.0142, -15.0275) (-86.0078, -15.0742) (-86.0011, -15.1209) (-85.9942, -15.1677) (-85.9869, -15.2145) (-85.9794, -15.2613) (-85.9716, -15.3082) (-85.9635, -15.3551) (-85.9551, -15.4021) (-85.9465, -15.4491) (-85.9376, -15.4961) (-85.9284, -15.5431) (-85.9189, -15.5902) (-85.9092, -15.6373) (-85.8992, -15.6845) (-85.8889, -15.7316) (-85.8784, -15.7788) (-85.8676, -15.826) (-85.8566, -15.8732) (-85.8475, -15.911) (-85.8406, -15.9394) (-85.8359, -15.9583) (-85.8336, -15.9678) knots 0 0 0 0 0 0 0.01428571 0.02857143 0.04285714 0.05714286 0.07142857 0.08571429 0.1 0.11428571 0.12857143 0.14285714 0.15714286 0.17142857 0.18571429 0.2 0.21428571 0.22857143 0.24285714 0.25714286 0.27142857 0.28571429 0.3 0.31428571 0.32857143 0.34285714 0.35714286 0.37142857 0.38571429 0.4 0.41428571 0.42857143 0.44285714 0.45714286 0.47142857 0.48571429 0.5 0.51428571 0.52857143 0.54285714 0.55714286 0.57142857 0.58571429 0.6 0.61428571 0.62857143 0.64285714 0.65714286 0.67142857 0.68571429 0.7 0.71428571 0.72857143 0.74285714 0.75714286 0.77142857 0.78571429 0.8 0.81428571 0.82857143 0.84285714 0.85714286 0.87142857 0.88571429 0.9 0.91428571 0.92857143 0.94285714 0.95714286 0.97142857 0.98571429 1 1 1 1 1 1
  arc A37 (-85.8336, -15.9678) -> (-84.6661, -16.3471) centre (-80, 0) ccw
  spline S7 degree 5 poles (-84.6661, -16.3471) (-84.6587, -16.3408) (-84.6438, -16.3283) (-84.6215, -16.3094) (-84.592, -16.2841) (-84.5553, -16.2524) (-84.5188, -16.2206) (-84.4826, -16.1886) (-84.4465, -16.1565) (-84.4107, -16.1242) (-84.3752, -16.0918) (-84.3399, -16.0593) (-84.3048, -16.0266) (-84.2699, -15.9938) (-84.2353, -15.9609) (-84.201, -15.9278) (-84.1668, -15.8946) (-84.133, -15.8613) (-84.0993, -15.8278) (-84.066, -15.7942) (-84.0328, -15.7604) (-84, -15.7266) (-83.9673, -15.6926) (-83.935, -15.6584) (-83.9029, -15.6242) (-83.8711, -15.5898) (-83.8395, -15.5552) (-83.8082, -15.5206) (-83.7772, -15.4858) (-83.7464, -15.4509) (-83.716, -15.4158) (-83.6858, -15.3806) (-83.6559, -15.3453) (-83.6263, -15.3099) (-83.5969, -15.2743) (-83.5679, -15.2386) (-83.5391, -15.2028) (-83.5107, -15.1668) (-83.4825, -15.1308) (-83.4547, -15.0945) (-83.4272, -15.0582) (-83.3999, -15.0217) (-83.3731, -14.9851) (-83.3465, -14.9484) (-83.3203, -14.9116) (-83.2944, -14.8746) (-83.2688, -14.8375) (-83.2435, -14.8002) (-83.2186, -14.7629) (-83.1941, -14.7254) (-83.1699, -14.6877) (-83.1461, -14.65) (-83.1228, -14.6121) (-83.0998, -14.574) (-83.0772, -14.5358) (-83.0551, -14.4975) (-83.0333, -14.4591) (-83.0118, -14.4205) (-82.9907, -14.3819) (-82.9701, -14.3431) (-82.95, -14.3041) (-82.9305, -14.2649) (-82.9117, -14.2256) (-82.8935, -14.1861) (-82.8759, -14.1464) (-82.8588, -14.1065) (-82.8419, -14.0666) (-82.8254, -14.0267) (-82.8094, -13.9866) (-82.7942, -13.9463) (-82.7804, -13.9057) (-82.7708, -13.8728) (-82.7646, -13.8478) (-82.761, -13.8311) (-82.7594, -13.8227) knots -1 -1 -1 -1 -1 -1 -0.98571429 -0.97142857 -0.95714286 -0.94285714 -0.92857143 -0.91428571 -0.9 -0.88571429 -0.87142857 -0.85714286 -0.84285714 -0.82857143 -0.81428571 -0.8 -0.78571429 -0.77142857 -0.75714286 -0.74285714 -0.72857143 -0.71428571 -0.7 -0.68571429 -0.67142857 -0.65714286 -0.64285714 -0.62857143 -0.61428571 -0.6 -0.58571429 -0.57142857 -0.55714286 -0.54285714 -0.52857143 -0.51428571 -0.5 -0.48571429 -0.47142857 -0.45714286 -0.44285714 -0.42857143 -0.41428571 -0.4 -0.38571429 -0.37142857 -0.35714286 -0.34285714 -0.32857143 -0.31428571 -0.3 -0.28571429 -0.27142857 -0.25714286 -0.24285714 -0.22857143 -0.21428571 -0.2 -0.18571429 -0.17142857 -0.15714286 -0.14285714 -0.12857143 -0.11428571 -0.1 -0.08571429 -0.07142857 -0.05714286 -0.04285714 -0.02857143 -0.01428571 0 0 0 0 0 0
  arc A38 (-81.5413, -12.4542) -> (-81.0818, -12.5025) centre (-80, 0) ccw
  spline S8 degree 5 poles (-80.1748, -14.0943) (-80.1749, -14.1029) (-80.1749, -14.12) (-80.1741, -14.1457) (-80.1716, -14.1799) (-80.1665, -14.2225) (-80.16, -14.2651) (-80.1526, -14.3076) (-80.1448, -14.3501) (-80.1366, -14.3927) (-80.1281, -14.4352) (-80.1192, -14.4777) (-80.1096, -14.5201) (-80.0994, -14.5625) (-80.0884, -14.6049) (-80.0769, -14.6471) (-80.0648, -14.6894) (-80.0522, -14.7316) (-80.0392, -14.7738) (-80.0259, -14.8159) (-80.0122, -14.858) (-79.998, -14.9) (-79.9835, -14.942) (-79.9685, -14.9839) (-79.9531, -15.0258) (-79.9373, -15.0677) (-79.9211, -15.1094) (-79.9045, -15.1512) (-79.8875, -15.1928) (-79.8702, -15.2345) (-79.8526, -15.276) (-79.8346, -15.3175) (-79.8162, -15.359) (-79.7975, -15.4004) (-79.7785, -15.4417) (-79.7591, -15.483) (-79.7394, -15.5242) (-79.7194, -15.5653) (-79.699, -15.6064) (-79.6784, -15.6474) (-79.6574, -15.6884) (-79.6361, -15.7293) (-79.6145, -15.7701) (-79.5926, -15.8109) (-79.5704, -15.8515) (-79.5478, -15.8922) (-79.525, -15.9327) (-79.5019, -15.9732) (-79.4785, -16.0136) (-79.4548, -16.0539) (-79.4308, -16.0942) (-79.4066, -16.1344) (-79.382, -16.1745) (-79.3572, -16.2145) (-79.3321, -16.2545) (-79.3067, -16.2944) (-79.281, -16.3342) (-79.2551, -16.3739) (-79.2289, -16.4136) (-79.2024, -16.4532) (-79.1757, -16.4927) (-79.1487, -16.5321) (-79.1214, -16.5714) (-79.0939, -16.6107) (-79.0661, -16.6498) (-79.0381, -16.6889) (-79.0098, -16.7279) (-78.9812, -16.7668) (-78.9524, -16.8056) (-78.9233, -16.8444) (-78.894, -16.883) (-78.8704, -16.9138) (-78.8525, -16.9369) (-78.8406, -16.9523) (-78.8346, -16.96) knots 0 0 0 0 0 0 0.01428571 0.02857143 0.04285714 0.05714286 0.07142857 0.08571429 0.1 0.11428571 0.12857143 0.14285714 0.15714286 0.17142857 0.18571429 0.2 0.21428571 0.22857143 0.24285714 0.25714286 0.27142857 0.28571429 0.3 0.31428571 0.32857143 0.34285714 0.35714286 0.37142857 0.38571429 0.4 0.41428571 0.42857143 0.44285714 0.45714286 0.47142857 0.48571429 0.5 0.51428571 0.52857143 0.54285714 0.55714286 0.57142857 0.58571429 0.6 0.61428571 0.62857143 0.64285714 0.65714286 0.67142857 0.68571429 0.7 0.71428571 0.72857143 0.74285714 0.75714286 0.77142857 0.78571429 0.8 0.81428571 0.82857143 0.84285714 0.85714286 0.87142857 0.88571429 0.9 0.91428571 0.92857143 0.94285714 0.95714286 0.97142857 0.98571429 1 1 1 1 1 1
  arc A39 (-78.8346, -16.96) -> (-77.6138, -16.8317) centre (-80, 0) ccw
  spline S9 degree 5 poles (-77.6138, -16.8317) (-77.6095, -16.8229) (-77.601, -16.8054) (-77.5884, -16.7791) (-77.5716, -16.744) (-77.551, -16.7001) (-77.5306, -16.6562) (-77.5105, -16.6122) (-77.4907, -16.5682) (-77.4711, -16.5242) (-77.4518, -16.4801) (-77.4328, -16.4361) (-77.414, -16.3919) (-77.3955, -16.3478) (-77.3773, -16.3036) (-77.3593, -16.2595) (-77.3417, -16.2152) (-77.3243, -16.171) (-77.3072, -16.1268) (-77.2904, -16.0825) (-77.2738, -16.0382) (-77.2576, -15.9939) (-77.2416, -15.9495) (-77.2259, -15.9052) (-77.2106, -15.8608) (-77.1955, -15.8165) (-77.1807, -15.7721) (-77.1662, -15.7277) (-77.152, -15.6833) (-77.1381, -15.6389) (-77.1245, -15.5945) (-77.1113, -15.5501) (-77.0983, -15.5056) (-77.0857, -15.4612) (-77.0733, -15.4168) (-77.0613, -15.3724) (-77.0496, -15.3279) (-77.0383, -15.2835) (-77.0272, -15.2391) (-77.0165, -15.1947) (-77.0061, -15.1503) (-76.9961, -15.1059) (-76.9864, -15.0616) (-76.9771, -15.0172) (-76.9681, -14.9729) (-76.9595, -14.9285) (-76.9512, -14.8842) (-76.9433, -14.8399) (-76.9358, -14.7957) (-76.9286, -14.7514) (-76.9218, -14.7072) (-76.9155, -14.6631) (-76.9095, -14.6189) (-76.904, -14.5748) (-76.8989, -14.5308) (-76.8943, -14.4867) (-76.89, -14.4428) (-76.8861, -14.3988) (-76.8825, -14.3549) (-76.8795, -14.3111) (-76.877, -14.2673) (-76.8751, -14.2236) (-76.8739, -14.18) (-76.8734, -14.1365) (-76.8734, -14.0931) (-76.874, -14.0497) (-76.8748, -14.0064) (-76.876, -13.9632) (-76.8776, -13.9201) (-76.8801, -13.8771) (-76.884, -13.8343) (-76.8887, -13.8004) (-76.8932, -13.7751) (-76.8967, -13.7583) (-76.8986, -13.75) knots -1 -1 -1 -1 -1 -1 -0.98571429 -0.97142857 -0.95714286 -0.94285714 -0.92857143 -0.91428571 -0.9 -0.88571429 -0.87142857 -0.85714286 -0.84285714 -0.82857143 -0.81428571 -0.8 -0.78571429 -0.77142857 -0.75714286 -0.74285714 -0.72857143 -0.71428571 -0.7 -0.68571429 -0.67142857 -0.65714286 -0.64285714 -0.62857143 -0.61428571 -0.6 -0.58571429 -0.57142857 -0.55714286 -0.54285714 -0.52857143 -0.51428571 -0.5 -0.48571429 -0.47142857 -0.45714286 -0.44285714 -0.42857143 -0.41428571 -0.4 -0.38571429 -0.37142857 -0.35714286 -0.34285714 -0.32857143 -0.31428571 -0.3 -0.28571429 -0.27142857 -0.25714286 -0.24285714 -0.22857143 -0.21428571 -0.2 -0.18571429 -0.17142857 -0.15714286 -0.14285714 -0.12857143 -0.11428571 -0.1 -0.08571429 -0.07142857 -0.05714286 -0.04285714 -0.02857143 -0.01428571 0 0 0 0 0 0
  arc A40 (-76.3425, -12.0044) -> (-75.903, -11.8616) centre (-80, 0) ccw
  spline S10 degree 5 poles (-74.4271, -12.9469) (-74.4237, -12.9548) (-74.4166, -12.9704) (-74.4054, -12.9935) (-74.3893, -13.0237) (-74.3673, -13.0606) (-74.344, -13.0969) (-74.32, -13.1327) (-74.2956, -13.1684) (-74.2708, -13.2039) (-74.2457, -13.2393) (-74.2203, -13.2745) (-74.1943, -13.3094) (-74.1677, -13.3439) (-74.1405, -13.3782) (-74.1127, -13.4121) (-74.0845, -13.4458) (-74.0558, -13.4792) (-74.0268, -13.5125) (-73.9975, -13.5455) (-73.9678, -13.5784) (-73.9378, -13.611) (-73.9075, -13.6435) (-73.8767, -13.6757) (-73.8456, -13.7077) (-73.8141, -13.7395) (-73.7823, -13.7711) (-73.7502, -13.8024) (-73.7178, -13.8336) (-73.685, -13.8646) (-73.652, -13.8954) (-73.6187, -13.926) (-73.5851, -13.9564) (-73.5512, -13.9866) (-73.517, -14.0166) (-73.4825, -14.0464) (-73.4477, -14.0761) (-73.4127, -14.1055) (-73.3774, -14.1348) (-73.3418, -14.1638) (-73.306, -14.1927) (-73.2699, -14.2214) (-73.2335, -14.2499) (-73.1969, -14.2782) (-73.1601, -14.3063) (-73.123, -14.3343) (-73.0857, -14.3621) (-73.0481, -14.3896) (-73.0103, -14.417) (-72.9722, -14.4443) (-72.9339, -14.4713) (-72.8954, -14.4981) (-72.8567, -14.5248) (-72.8177, -14.5513) (-72.7785, -14.5776) (-72.7391, -14.6037) (-72.6995, -14.6296) (-72.6596, -14.6554) (-72.6196, -14.6809) (-72.5793, -14.7063) (-72.5388, -14.7315) (-72.4981, -14.7565) (-72.4572, -14.7814) (-72.4161, -14.806) (-72.3748, -14.8305) (-72.3332, -14.8548) (-72.2915, -14.8789) (-72.2496, -14.9028) (-72.2075, -14.9266) (-72.1652, -14.9502) (-72.1227, -14.9735) (-72.0885, -14.9921) (-72.0628, -15.0059) (-72.0457, -15.0151) (-72.0371, -15.0197) knots 0 0 0 0 0 0 0.01428571 0.02857143 0.04285714 0.05714286 0.07142857 0.08571429 0.1 0.11428571 0.12857143 0.14285714 0.15714286 0.17142857 0.18571429 0.2 0.21428571 0.22857143 0.24285714 0.25714286 0.27142857 0.28571429 0.3 0.31428571 0.32857143 0.34285714 0.35714286 0.37142857 0.38571429 0.4 0.41428571 0.42857143 0.44285714 0.45714286 0.47142857 0.48571429 0.5 0.51428571 0.52857143 0.54285714 0.55714286 0.57142857 0.58571429 0.6 0.61428571 0.62857143 0.64285714 0.65714286 0.67142857 0.68571429 0.7 0.71428571 0.72857143 0.74285714 0.75714286 0.77142857 0.78571429 0.8 0.81428571 0.82857143 0.84285714 0.85714286 0.87142857 0.88571429 0.9 0.91428571 0.92857143 0.94285714 0.95714286 0.97142857 0.98571429 1 1 1 1 1 1
  arc A41 (-72.0371, -15.0197) -> (-70.974, -14.406) centre (-80, 0) ccw
  spline S11 degree 5 poles (-70.974, -14.406) (-70.9737, -14.3962) (-70.9731, -14.3768) (-70.9722, -14.3476) (-70.9712, -14.3087) (-70.9702, -14.2602) (-70.9694, -14.2118) (-70.969, -14.1635) (-70.9687, -14.1152) (-70.9687, -14.067) (-70.969, -14.0189) (-70.9696, -13.9709) (-70.9704, -13.923) (-70.9714, -13.8751) (-70.9727, -13.8274) (-70.9743, -13.7797) (-70.9762, -13.7321) (-70.9783, -13.6846) (-70.9806, -13.6373) (-70.9833, -13.59) (-70.9862, -13.5428) (-70.9894, -13.4957) (-70.9928, -13.4487) (-70.9965, -13.4018) (-71.0005, -13.355) (-71.0048, -13.3084) (-71.0093, -13.2618) (-71.0142, -13.2154) (-71.0193, -13.169) (-71.0246, -13.1228) (-71.0303, -13.0767) (-71.0362, -13.0307) (-71.0425, -12.9849) (-71.049, -12.9391) (-71.0558, -12.8935) (-71.0629, -12.8481) (-71.0703, -12.8027) (-71.0779, -12.7575) (-71.0859, -12.7125) (-71.0942, -12.6676) (-71.1028, -12.6228) (-71.1117, -12.5782) (-71.1209, -12.5337) (-71.1304, -12.4894) (-71.1402, -12.4452) (-71.1504, -12.4012) (-71.1609, -12.3574) (-71.1717, -12.3137) (-71.1828, -12.2702) (-71.1942, -12.2269) (-71.206, -12.1837) (-71.2181, -12.1408) (-71.2307, -12.098) (-71.2436, -12.0555) (-71.2569, -12.0132) (-71.2705, -11.9711) (-71.2844, -11.9292) (-71.2987, -11.8874) (-71.3134, -11.8459) (-71.3284, -11.8046) (-71.3439, -11.7636) (-71.36, -11.7229) (-71.3766, -11.6826) (-71.3939, -11.6426) (-71.4116, -11.603) (-71.4297, -11.5636) (-71.4481, -11.5244) (-71.4667, -11.4854) (-71.4858, -11.4466) (-71.5055, -11.4084) (-71.5265, -11.3709) (-71.5445, -11.3418) (-71.559, -11.3205) (-71.569, -11.3066) (-71.5741, -11.2998) knots -1 -1 -1 -1 -1 -1 -0.98571429 -0.97142857 -0.95714286 -0.94285714 -0.92857143 -0.91428571 -0.9 -0.88571429 -0.87142857 -0.85714286 -0.84285714 -0.82857143 -0.81428571 -0.8 -0.78571429 -0.77142857 -0.75714286 -0.74285714 -0.72857143 -0.71428571 -0.7 -0.68571429 -0.67142857 -0.65714286 -0.64285714 -0.62857143 -0.61428571 -0.6 -0.58571429 -0.57142857 -0.55714286 -0.54285714 -0.52857143 -0.51428571 -0.5 -0.48571429 -0.47142857 -0.45714286 -0.44285714 -0.42857143 -0.41428571 -0.4 -0.38571429 -0.37142857 -0.35714286 -0.34285714 -0.32857143 -0.31428571 -0.3 -0.28571429 -0.27142857 -0.25714286 -0.24285714 -0.22857143 -0.21428571 -0.2 -0.18571429 -0.17142857 -0.15714286 -0.14285714 -0.12857143 -0.11428571 -0.1 -0.08571429 -0.07142857 -0.05714286 -0.04285714 -0.02857143 -0.01428571 0 0 0 0 0 0
  arc A42 (-71.7761, -9.4789) -> (-71.4327, -9.1697) centre (-80, 0) ccw
  spline S12 degree 5 poles (-69.6429, -9.5609) (-69.6366, -9.5667) (-69.6238, -9.5781) (-69.6042, -9.5947) (-69.5771, -9.6157) (-69.542, -9.6404) (-69.506, -9.6641) (-69.4695, -9.6871) (-69.4327, -9.7097) (-69.3956, -9.7321) (-69.3583, -9.7542) (-69.3207, -9.776) (-69.2828, -9.7973) (-69.2444, -9.8181) (-69.2057, -9.8383) (-69.1665, -9.858) (-69.127, -9.8773) (-69.0872, -9.8962) (-69.0472, -9.9147) (-69.007, -9.933) (-68.9665, -9.951) (-68.9258, -9.9686) (-68.8849, -9.9859) (-68.8437, -10.0028) (-68.8022, -10.0194) (-68.7606, -10.0356) (-68.7187, -10.0515) (-68.6766, -10.0671) (-68.6343, -10.0824) (-68.5918, -10.0974) (-68.5491, -10.1121) (-68.5062, -10.1265) (-68.4631, -10.1406) (-68.4198, -10.1544) (-68.3764, -10.1679) (-68.3327, -10.1811) (-68.2889, -10.1941) (-68.245, -10.2067) (-68.2008, -10.2191) (-68.1565, -10.2312) (-68.112, -10.243) (-68.0674, -10.2545) (-68.0226, -10.2658) (-67.9776, -10.2767) (-67.9325, -10.2875) (-67.8873, -10.2979) (-67.8419, -10.3081) (-67.7963, -10.318) (-67.7506, -10.3276) (-67.7048, -10.337) (-67.6588, -10.3461) (-67.6127, -10.355) (-67.5665, -10.3636) (-67.5201, -10.3719) (-67.4736, -10.38) (-67.427, -10.3879) (-67.3802, -10.3954) (-67.3334, -10.4027) (-67.2864, -10.4098) (-67.2392, -10.4166) (-67.192, -10.4232) (-67.1446, -10.4295) (-67.0972, -10.4355) (-67.0496, -10.4413) (-67.0019, -10.4469) (-66.9541, -10.4522) (-66.9061, -10.4572) (-66.8581, -10.4621) (-66.81, -10.4666) (-66.7618, -10.4709) (-66.7134, -10.475) (-66.6747, -10.4781) (-66.6456, -10.4803) (-66.6262, -10.4817) (-66.6164, -10.4824) knots 0 0 0 0 0 0 0.01428571 0.02857143 0.04285714 0.05714286 0.07142857 0.08571429 0.1 0.11428571 0.12857143 0.14285714 0.15714286 0.17142857 0.18571429 0.2 0.21428571 0.22857143 0.24285714 0.25714286 0.27142857 0.28571429 0.3 0.31428571 0.32857143 0.34285714 0.35714286 0.37142857 0.38571429 0.4 0.41428571 0.42857143 0.44285714 0.45714286 0.47142857 0.48571429 0.5 0.51428571 0.52857143 0.54285714 0.55714286 0.57142857 0.58571429 0.6 0.61428571 0.62857143 0.64285714 0.65714286 0.67142857 0.68571429 0.7 0.71428571 0.72857143 0.74285714 0.75714286 0.77142857 0.78571429 0.8 0.81428571 0.82857143 0.84285714 0.85714286 0.87142857 0.88571429 0.9 0.91428571 0.92857143 0.94285714 0.95714286 0.97142857 0.98571429 1 1 1 1 1 1
  arc A43 (-66.6164, -10.4824) -> (-65.8949, -9.4893) centre (-80, 0) ccw